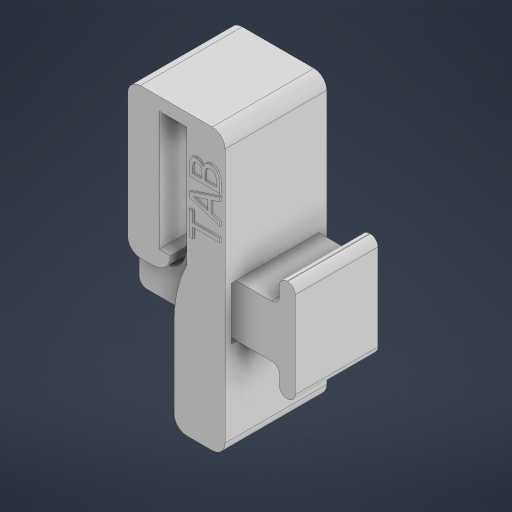
# Autodesk Inventor part: fet leg bender
Saved by Autodesk Inventor 2024.2 (Build 282272000, 272)
## iProperties
Created: 2023-11-28
Part Number: fet leg bender
Material: Generic
Document SubType Name: Modeling
Designer: voids
Density: 1 g/cm^3
Appearance: Default
Author: voids
Autodesk Inventor part; units mm, degrees
ref_plane "YZ Plane" through (0, 0, 0) normal (1, 0, 0) x (0, 1, 0)
ref_plane "XZ Plane" through (0, 0, 0) normal (0, 1, 0) x (-1, 0, 0)
ref_plane "XY Plane" through (0, 0, 0) normal (0, 0, 1) x (1, 0, 0)
sketch "Sketch1" plane through (0, 0, 0) normal (0, 0, 1) x (1, 0, 0)
  line L0 (0, 0) -> (5.461, 0)
  line L1 (5.461, 0) -> (5.461, 23.8506)
  line L2 (5.461, 23.8506) -> (0, 23.8506)
  line L3 (0, 23.8506) -> (0, 0)
  line L4 (-6.35, -3.4565) -> (-6.35, 26.3906)
  line L5 (-6.35, 26.3906) -> (13.081, 26.3906)
  line L6 (13.081, 26.3906) -> (13.081, 0)
  line L7 (6.2124, 5.3513) -> (6.2124, 12.7836) construction
  line L8 (6.2124, 12.7836) -> (9.1429, 12.7836) construction
  line L9 (9.1429, 12.7836) -> (9.1429, 5.3513) construction
  line L10 (9.1429, 5.3513) -> (6.2124, 5.3513) construction
  arc A0 (-1.2213, -3.4565) -> (2.2352, 0) centre (-1.2213, 0) ccw
  arc A1 (-1.2213, -4.1423) -> (2.921, 0) centre (-1.2213, 0) ccw
  line L11 (5.461, 17.5006) -> (0, 17.5006) construction
  line L12 (21.6327, -3.7994) -> (-20.9867, -3.7994) construction
  line L13 (-1.2213, -3.4565) -> (-1.2213, -4.1423) construction
  line L14 (-1.2213, -3.4565) -> (0.268, -3.4565)
  line L15 (0.268, -3.4565) -> (-6.35, -3.4565)
  line L16 (-1.2213, -4.1423) -> (-6.35, -4.1423)
  line L17 (-6.35, -4.1423) -> (-6.35, -16.8423)
  line L18 (-6.35, -10.4923) -> (13.081, -10.4923)
  line L19 (2.921, 0) -> (2.921, -16.8423) construction
  line L20 (2.921, -10.4923) -> (2.921, -11.9076)
  line L21 (13.081, 0) -> (5.461, 0)
  line L22 (-6.35, -16.8423) -> (13.081, -16.8423)
  line L23 (13.081, -16.8423) -> (13.081, 0)
  line L24 (13.081, 0) -> (23.241, 0)
  line L25 (23.241, 0) -> (23.241, -10.4923)
  line L26 (23.241, -10.4923) -> (13.081, -10.4923)
  line L27 (13.081, -10.4923) -> (13.081, 0)
  line L28 (-6.35, -10.4923) -> (-11.43, -10.4923)
  line L29 (-11.43, -10.4923) -> (-11.43, -4.1423)
  line L30 (-11.43, -4.1423) -> (-6.35, -4.1423)
  line L31 (-6.35, -4.1423) -> (-6.35, -10.4923)
  line L32 (2.921, 0) -> (2.921, -16.8423)
  line L33 (-6.35, -3.4565) -> (-6.35, -4.1423)
  line L34 (1.2228, -16.8423) -> (1.2228, -2.4441)
  line L35 (13.081, -16.8423) -> (2.921, -16.8423)
  line L36 (2.921, -16.8423) -> (2.921, -29.5423)
  line L37 (2.921, -29.5423) -> (13.081, -29.5423)
  line L38 (13.081, -29.5423) -> (13.081, -16.8423)
  line L39 (24.8285, -15.4062) -> (21.6535, -15.4062)
  line L40 (21.6535, -15.4062) -> (21.6535, 4.9138)
  line L41 (21.6535, 4.9138) -> (24.8285, 4.9138)
  line L42 (24.8285, 4.9138) -> (24.8285, -15.4062)
  line L43 (24.8285, -15.4062) -> (21.6535, 4.9138) construction
  line L44 (21.6535, -15.4062) -> (24.8285, 4.9138) construction
  line L45 (12.3084, 7.3916) -> (6.9337, 7.3916)
  line L46 (6.9337, 7.3916) -> (6.9337, 5.3464)
  line L47 (6.9337, 5.3464) -> (6.2124, 5.3464)
  line L48 (6.2124, 5.3464) -> (6.2124, 10.2469)
  line L49 (6.2124, 10.2469) -> (6.9337, 10.2469)
  line L50 (6.9337, 10.2469) -> (6.9337, 8.2017)
  line L51 (6.9337, 8.2017) -> (12.3084, 8.2017)
  line L52 (12.3084, 8.2017) -> (12.3084, 7.3916)
  line L53 (12.3084, 10.2074) -> (6.2124, 12.2625)
  line L54 (6.2124, 12.2625) -> (6.2124, 13.2603)
  line L55 (6.2124, 13.2603) -> (12.3084, 15.3154)
  line L56 (12.3084, 15.3154) -> (12.3084, 14.4608)
  line L57 (12.3084, 14.4608) -> (10.6041, 13.9075)
  line L58 (10.6041, 13.9075) -> (10.6041, 11.5807)
  line L59 (10.6041, 11.5807) -> (12.3084, 11.0274)
  line L60 (12.3084, 11.0274) -> (12.3084, 10.2074)
  line L61 (9.9125, 13.6852) -> (7.0424, 12.7416)
  line L62 (7.0424, 12.7416) -> (9.9125, 11.803)
  line L63 (9.9125, 11.803) -> (9.9125, 13.6852)
  spline S0 degree 2 poles (10.4362, 20.0282) (10.8907, 20.0282) (11.5872, 19.6824) (11.8144, 19.3959) knots 0 0 0 1 2 2 2
  spline S1 degree 2 poles (11.8144, 19.3959) (12.0812, 19.0501) (12.3084, 18.2646) (12.3084, 17.6421) knots 0 0 0 1 2 2 2
  line L64 (12.3084, 17.6421) -> (12.3084, 15.8934)
  line L65 (12.3084, 15.8934) -> (6.2124, 15.8934)
  line L66 (6.2124, 15.8934) -> (6.2124, 17.5088)
  spline S2 degree 2 poles (6.2124, 17.5088) (6.2124, 18.1609) (6.2964, 18.8129) (6.4594, 19.1093) knots 0 0 0 1 2 2 2
  spline S3 degree 2 poles (6.4594, 19.1093) (6.6323, 19.4403) (7.2004, 19.7417) (7.5858, 19.7417) knots 0 0 0 1 2 2 2
  spline S4 degree 2 poles (7.5858, 19.7417) (8.0156, 19.7417) (8.6973, 19.2872) (8.8899, 18.887) knots 0 0 0 1 2 2 2
  line L67 (8.8899, 18.887) -> (8.9196, 18.887)
  spline S5 degree 2 poles (8.9196, 18.887) (9.0678, 19.4304) (9.8532, 20.0282) (10.4362, 20.0282) knots 0 0 0 1 2 2 2
  spline S6 degree 2 poles (10.4707, 19.1834) (10.1249, 19.1834) (9.6803, 18.9858) (9.5223, 18.6894) knots 0 0 0 1 2 2 2
  spline S7 degree 2 poles (9.5223, 18.6894) (9.4235, 18.4968) (9.3642, 18.0423) (9.3642, 17.6224) knots 0 0 0 1 2 2 2
  line L68 (9.3642, 17.6224) -> (9.3642, 16.7035)
  line L69 (9.3642, 16.7035) -> (11.6168, 16.7035)
  line L70 (11.6168, 16.7035) -> (11.6168, 17.3606)
  spline S8 degree 2 poles (11.6168, 17.3606) (11.6168, 17.8941) (11.518, 18.5067) (11.36, 18.7438) knots 0 0 0 1 2 2 2
  spline S9 degree 2 poles (11.36, 18.7438) (11.1969, 18.971) (10.7919, 19.1834) (10.4707, 19.1834) knots 0 0 0 1 2 2 2
  spline S10 degree 2 poles (7.6994, 18.8969) (7.482, 18.8969) (7.156, 18.7487) (7.0621, 18.5857) knots 0 0 0 1 2 2 2
  spline S11 degree 2 poles (7.0621, 18.5857) (6.9534, 18.3881) (6.904, 17.9089) (6.904, 17.4791) knots 0 0 0 1 2 2 2
  line L71 (6.904, 17.4791) -> (6.904, 16.7035)
  line L72 (6.904, 16.7035) -> (8.6874, 16.7035)
  line L73 (8.6874, 16.7035) -> (8.6874, 17.6224)
  spline S12 degree 2 poles (8.6874, 17.6224) (8.6874, 18.0028) (8.6084, 18.3634) (8.4849, 18.5561) knots 0 0 0 1 2 2 2
  spline S13 degree 2 poles (8.4849, 18.5561) (8.3663, 18.7438) (7.9859, 18.8969) (7.6994, 18.8969) knots 0 0 0 1 2 2 2
  point P0 (-1.2213, -3.7994)
  point P1 (13.081, -10.4923)
  point P2 (-6.35, -4.1423)
  point P3 (2.921, -10.4923)
  point P4 (2.921, -16.8423)
  point P5 (23.241, -5.2462)
  point P6 (21.6535, -10.4923)
  point P7 (21.6535, 0)
  dimension "d0" = 5.461
  dimension "d1" = 23.8506
  dimension "d2" = 0.6858
  dimension "d3" = 2.54
  dimension "d4" = 21.3
  dimension "d5" = 6.35
  dimension "d8" = 5.8581
  dimension "d9" = -1.4893
  dimension "d10" = 6.35
  dimension "d11" = 6.35
  dimension "d12" = 2.54
  dimension "d13" = 6.35
  dimension "d14" = 7.62
  dimension "d15" = 5.08
  dimension "d16" = 10.16
  dimension "d25" = 1.6982
  dimension "d28" = 12.7
  dimension "d36" = 3.175
  dimension "d37" = 20.32
  constraints: 82 end point, 13 point on line, 11 parallel, 11 perpendicular, 10 horizontal, 6 collinear, 5 midpoint, 5 point on circle, 2 centre point, 2 line through centre, 2 vertical, 3 other
  measures "d0" distance of L2.end L1.end
  measures "d1" distance of L0.end L1.end
  measures "d2" radial gap between concentric circles of A0 A1
  measures "d3" distance from line of L19.start L1
  measures "d4" distance between parallel lines of L12 L11
  measures "d5" distance between parallel lines of L2 L11
  measures "d8" distance of L19.start L13.end
  measures "d9" distance of L13.start L14.end
  measures "d10" distance between parallel lines of L3 L4
  measures "d11" distance between parallel lines of L16 L18
  measures "d12" distance between parallel lines of L5 L2
  measures "d13" distance from line of L17.end L18
  measures "d14" distance between parallel lines of L1 L6
  measures "d15" distance of L29.end L30.end
  measures "d16" distance of L25.end L26.end
  measures "d25" distance between parallel lines of L32 L34
  measures "d28" distance of L36.end L35.end
  measures "d36" distance of L40.end L41.end
  measures "d37" distance of L39.end L40.end
extrude "Extrusion1" add sketch "Sketch1" against normal blind 1.524 contours L3 L2 L1 L0 | L0 A0 L15 L4 L5 L6 L21 L1 L2 L3 | L0 A1 L34 A0 | L32 L18 L34 A1 | L0 L21 L23 L18 L32 | L34 A1 L16 L33 L15 A0 | L34 L18 L17 L16 A1 | L20 L32 L22 L34 L18 | L18 L23 L22 L32 L20 | L34 L22 L17 L18 | L38 L37 L36 L22 | L45 L46 L47 L48 L49 L50 L51 L52 | L53 L54 L55 L56 L57 L58 L59 L60 | L63 L62 L61 | S0 S1 L64 L65 L66 S2 S3 S4 L67 S5 | S9 S8 L70 L69 L68 S7 S6 | S13 S12 L73 L72 L71 S11 S10
extrude "Extrusion2" add sketch "Sketch1" along normal blind 1.27 contours L3 L2 L1 L0 | L0 A0 L15 L4 L5 L6 L21 L1 L2 L3 | L20 L32 L22 L34 L18 | L18 L23 L22 L32 L20 | L34 L22 L17 L18 | L38 L37 L36 L22 | L45 L46 L47 L48 L49 L50 L51 L52 | L53 L54 L55 L56 L57 L58 L59 L60 | L63 L62 L61 | S0 S1 L64 L65 L66 S2 S3 S4 L67 S5 | S9 S8 L70 L69 L68 S7 S6 | S13 S12 L73 L72 L71 S11 S10
extrude "Extrusion3" add sketch "Sketch1" along normal blind 16.256 from surface at 1.27 contours L0 A0 L15 L4 L5 L6 L21 L1 L2 L3 | L18 L23 L22 L32 L20 | L38 L37 L36 L22 | L45 L46 L47 L48 L49 L50 L51 L52 | L53 L54 L55 L56 L57 L58 L59 L60 | L63 L62 L61 | S0 S1 L64 L65 L66 S2 S3 S4 L67 S5 | S9 S8 L70 L69 L68 S7 S6 | S13 S12 L73 L72 L71 S11 S10
extrude "Extrusion4" add sketch "Sketch1" along normal blind 1.27 from surface at 17.526 contours L0 A0 L15 L4 L5 L6 L21 L1 L2 L3 | L0 L21 L23 L18 L32 | L18 L23 L22 L32 L20 | L38 L37 L36 L22 | L45 L46 L47 L48 L49 L50 L51 L52 | L53 L54 L55 L56 L57 L58 L59 L60 | L63 L62 L61 | S0 S1 L64 L65 L66 S2 S3 S4 L67 S5 | S9 S8 L70 L69 L68 S7 S6 | S13 S12 L73 L72 L71 S11 S10
extrude "Extrusion5" add sketch "Sketch1" along normal blind 16.51 separate body contours L32 L18 L34 A1 | L0 L21 L23 L18 L32 | L34 L18 L17 L16 A1 | L24 L40 L26 L23 | L40 L41 L42 L39 L26 L25 L24 | L24 L25 L26 L40
extrude "Extrusion6" add sketch "Sketch1" along normal blind 0.254 from surface at 18.796 contours L45 L46 L47 L48 L49 L50 L51 L52 | L53 L54 L55 L56 L57 L58 L59 L60 | S0 S1 L64 L65 L66 S2 S3 S4 L67 S5 bodies 1
thicken "Thicken1" operation cut thickness 0.0508 both sides no extend neighbours no toward (0, 1, 0) bodies 2 faces at (2.9845, -10.4923, 5.5033)
thicken "Thicken2" operation cut thickness 0.0508 both sides no extend neighbours no toward (0, -1, 0) bodies 2 faces at (15.4093, 0, 5.5033) (0.2921, -3.856, 11.0067) (-2.9309, -4.1423, 5.5033)
fillet "Fillet1" radius 25.4 1 edges at (2.921, 0, 18.161)
fillet "Fillet2" radius 1.524 6 edges at (21.6535, -0.0508, 8.255) (21.6535, 4.9138, 8.255) (24.8285, 4.9138, 8.255) (21.6535, -10.4415, 8.255) (21.6535, -15.4062, 8.255) (24.8285, -15.4062, 8.255)
fillet "Fillet3" radius 1.524 2 edges at (-6.35, -10.4415, 8.255) (-6.35, -4.1931, 8.255)
fillet "Fillet4" radius 2.54 8 edges at (13.081, -29.5423, 8.636) (2.921, -29.5423, 8.636) (-6.35, -16.8423, -0.127) (2.921, -16.8423, -0.127) (-6.35, 26.3906, 8.636) (-6.35, -3.4565, 0.635) (-6.35, -3.4565, 10.033) (13.081, 26.3906, 8.636)
body "Solid1"
body "Solid2"
